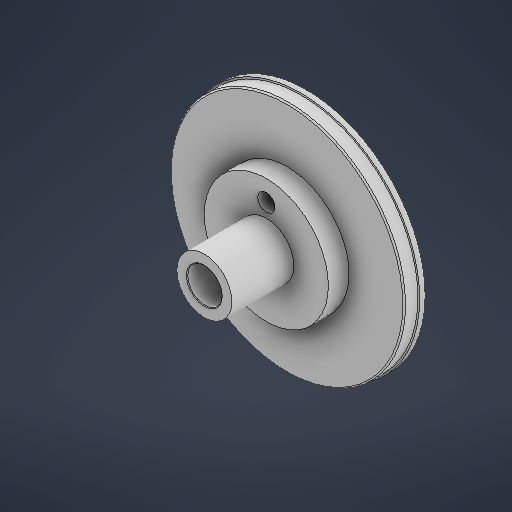
# Autodesk Inventor part: HeatExchangePistonExhaust
Saved by Autodesk Inventor 2025.4 (Build 294407000, 407)
## iProperties
Created: 2026-05-29
Part Number: HeatExchangePistonExhaust
Material: Generic
Document SubType Name: Modeling
Designer: VuQuan
Density: 1 g/cm^3
Appearance: Default
Author: VuQuan
Autodesk Inventor part; units mm, degrees
ref_plane "YZ Plane" through (0, 0, 0) normal (1, 0, 0) x (0, 1, 0)
ref_plane "XZ Plane" through (0, 0, 0) normal (0, 1, 0) x (-1, 0, 0)
ref_plane "XY Plane" through (0, 0, 0) normal (0, 0, 1) x (1, 0, 0)
sketch "Sketch1" plane through (0, 0, 0) normal (0, 0, 1) x (1, 0, 0)
  circle A0 centre (0, 0) radius 17
  circle A1 centre (0, 0) radius 17.25
  circle A2 centre (0, 0) radius 4
  circle A3 centre (0, 0) radius 9
  circle A4 centre (0, 0) radius 2.5
  circle A5 centre (0, 6) radius 1.25
  dimension "d0" = 34
  dimension "d1" = 34.5
  dimension "d2" = 8
  dimension "d3" = 18
  dimension "d4" = 5
  dimension "d5" = 2.5
  dimension "d6" = 6
  constraints: 6 centre point, 5 coincident, 1 vertical alignment
  measures "d0" diameter of A0
  measures "d1" diameter of A1
  measures "d2" diameter of A2
  measures "d3" diameter of A3
  measures "d4" diameter of A4
  measures "d5" diameter of A5
  measures "d6" distance of A5.centre point (0, 0)
extrude "Extrusion1" add sketch "Sketch1" along normal blind 1 contours A1
extrude "Extrusion2" add sketch "Sketch1" along normal blind 3 contours A0
extrude "Extrusion3" add sketch "Sketch1" along normal blind 6 contours A3
extrude "Extrusion4" add sketch "Sketch1" along normal blind 15 contours A2
chamfer "Chamfer1" distance 0.2 angle 45 2 edges at (-17.25, 0, 0) (-17, 0, 3)
chamfer "Chamfer2" distance 0.1 angle 45 1 edges at (-2.5, 0, 15)
body "Solid1"
